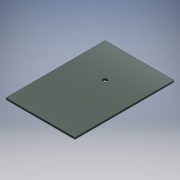
# Autodesk Inventor part: base
Saved by Autodesk Inventor 2016 (Build 200138000, 138)
## iProperties
Created: 2016-09-20
Part Number: base
Material: Madera (abedul)
Document SubType Name: Modeling
Designer: i95sa
Density: 0.55 g/cm^3
Appearance: Gris plomo - Pulido
Author: i95sa
Autodesk Inventor part; units mm, degrees
ref_plane "YZ Plane" through (0, 0, 0) normal (1, 0, 0) x (0, 1, 0)
ref_plane "XZ Plane" through (0, 0, 0) normal (0, 1, 0) x (-1, 0, 0)
ref_plane "XY Plane" through (0, 0, 0) normal (0, 0, 1) x (1, 0, 0)
sketch "Boceto1" plane through (0, 0, 0) normal (0, 0, 1) x (1, 0, 0)
  circle A0 centre (0, 0) radius 5
  line L0 (0, 0) -> (0, -150)
  line L1 (0, 0) -> (0, 80)
  line L2 (0, 80) -> (80, 80)
  line L3 (80, 80) -> (80, -150)
  line L4 (80, -150) -> (-80, -150)
  line L5 (-80, -150) -> (-80, 80)
  line L6 (-80, 80) -> (0, 80)
  dimension "d0" = 10
  dimension "d1" = 150
  dimension "d2" = 80
  dimension "d3" = 80
  dimension "d4" = 160
  constraints: 14 end point, 5 perpendicular, 2 vertical, 1 centre point, 1 coincident, 1 point on line
  measures "d0" diameter of A0
  measures "d1" distance of L0.start L0.end
  measures "d2" distance of L0.start L1.end
  measures "d3" distance of L1.end L2.end
  measures "d4" distance of L3.end L4.end
extrude "Extrusión1" add sketch "Boceto1" along normal blind 4 contours A0 L1 L2 L3 L4 L0 | A0 L0 L4 L5 L6 L1
